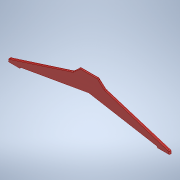
# Autodesk Inventor part: ramínko
Saved by Autodesk Inventor 2021.3 (Build 253353000, 353)
## iProperties
Created: 2021-05-28
Part Number: ramínko
Material: Všeobecné
Document SubType Name: Modeling
Designer: honza
Density: 1 g/cm^3
Appearance: Oranžovo-červená
Author: honza
Autodesk Inventor part; units mm, degrees
ref_plane "YZ Plane" through (0, 0, 0) normal (1, 0, 0) x (0, 1, 0)
ref_plane "XZ Plane" through (0, 0, 0) normal (0, 1, 0) x (-1, 0, 0)
ref_plane "XY Plane" through (0, 0, 0) normal (0, 0, 1) x (1, 0, 0)
sketch "Náčrt1" plane through (0, 0, 0) normal (0, 0, 1) x (1, 0, 0)
  arc A0 (204.9384, 11.1978) -> (199.6186, 15.4008) centre (200, 10.4153) ccw
  line L0 (204.9384, 11.1978) -> (240, 11.1978)
  line L1 (240, 11.1978) -> (239.8691, 16.1961)
  line L2 (240, 11.1978) -> (245, 11.1978) construction
  line L3 (0, 0) -> (0, 101.1978)
  arc A1 (29.5004, 98.3765) -> (25, 101.1978) centre (25, 96.1978) ccw
  arc A2 (46.6016, 82.5302) -> (50, 81.1978) centre (50, 86.1978) ccw
  line L4 (25, 101.1978) -> (0, 101.1978)
  line L5 (29.5004, 98.3765) -> (46.6016, 82.5302)
  line L6 (50, 81.1978) -> (234.8691, 21.1961)
  line L7 (0, 50.5989) -> (199.6186, 15.4008)
  arc A3 (234.7382, 11.1978) -> (235, 11.1978) centre (234.8691, 16.1961) ccw
  arc A4 (239.8691, 16.1961) -> (234.8691, 21.1961) centre (234.8691, 16.1961) ccw
  dimension "d0" = 10
  dimension "d1" = 200
  dimension "d8" = 240
  dimension "d9" = 5
  dimension "d10" = 91.5
  dimension "d13" = 90
  dimension "d14" = 10
  dimension "d15" = 25
  dimension "d17" = 10
  dimension "d18" = 50
  dimension "d20" = 155.163
  dimension "d21" = 80
  constraints: 16 end point, 10 point on circle, 5 centre point, 3 horizontal, 2 point on line, 2 tangent, 1 equal length, 1 midpoint, 1 vertical
  measures "d0" diameter of A0
  measures "d1" horizontal distance of L3.start A0.centre
  measures "d8" horizontal distance of L3.start L0.end
  measures "d9" distance of L0.end L1.end
  measures "d10" angle of L2 L1
  measures "d13" vertical distance of L0.end L3.end
  measures "d14" diameter of A1
  measures "d15" distance from line of L3 A1.centre
  measures "d17" diameter of A2
  measures "d18" distance from line of L3 A2.centre
  measures "d20" angle of L5 L6
  measures "d21" angle of L7 L3
sketch "Náčrt2" plane through (0, 0, 0) normal (0, 1, 0) x (-1, 0, 0)
  line L0 (240, -7.5) -> (-240, -7.5)
  line L1 (-240, -7.5) -> (-240, 7.5)
  line L2 (-240, 7.5) -> (240, 7.5)
  line L3 (240, 7.5) -> (240, -7.5)
  line L4 (240, -7.5) -> (-240, 7.5) construction
  line L5 (-240, -7.5) -> (240, 7.5) construction
  point P0 (0, 0)
  dimension "d22" = 480
  dimension "d23" = 15
  constraints: 12 end point, 2 midpoint, 2 parallel, 1 horizontal, 1 perpendicular
  measures "d22" distance of L1.end L2.end
  measures "d23" distance of L0.end L1.end
extrude "Vysunutí1" add sketch "Náčrt2" along normal up to surface (101.1978 mm away) draft -1.5
extrude "Vysunutí2" cut sketch "Náčrt1" against normal blind 10 keep common part
shell "Skořepina1" thickness 1 removed faces 4 at (0, 67.4652, -3.675) at (133.079, 27.1335, -4.4239) at (204.8568, 11.6034, -4.7941) at (228.1173, 11.1978, -4.8045)
fillet "Zaoblení1" radius 2 12 edges at (27.6558, 100.4341, -4.87) (27.6558, 100.4341, 0) (48.1749, 81.5428, 0) (38.051, 90.4534, 0) (48.1749, 81.5428, -5.3647) (38.051, 90.4534, -5.1314) (142.4346, 51.1969, -6.1594) (142.4346, 51.1969, 0) (237.6913, 20.3235, 0) (237.6913, 20.3235, -6.9678) (239.6176, 14.604, 0) (239.6176, 14.604, -7.1176)
mirror "Zrcadlit1" about plane through (0, 0, 0) normal (1, 0, 0)
